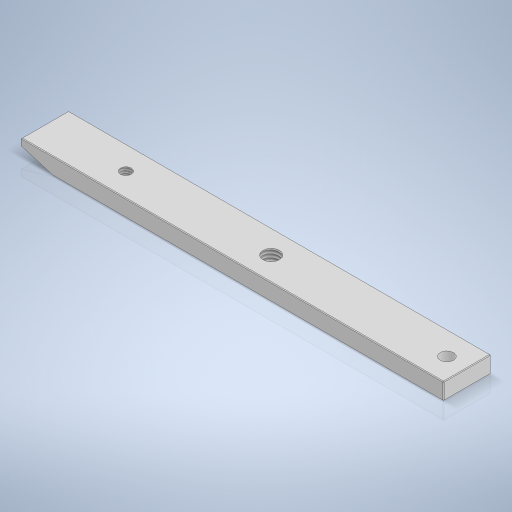
# Autodesk Inventor part: 112
Saved by Autodesk Inventor 2024 (Build 280153000, 153)
## iProperties
Created: 2024-06-07
Part Number: 112
Material: Generisch
Document SubType Name: Modeling
Designer: ffogue
Density: 1 g/cm^3
Appearance: Vorgabe
Author: ffogue
Autodesk Inventor part; units mm, degrees
ref_plane "YZ Plane" through (0, 0, 0) normal (1, 0, 0) x (0, 1, 0)
ref_plane "XZ Plane" through (0, 0, 0) normal (0, 1, 0) x (-1, 0, 0)
ref_plane "XY Plane" through (0, 0, 0) normal (0, 0, 1) x (1, 0, 0)
sketch "Skizze1" plane through (0, 0, 0) normal (0, 1, 0) x (-1, 0, 0)
  line L0 (0, 3) -> (0, 5)
  line L1 (0, 5) -> (-125, 5)
  line L2 (-125, 5) -> (-125, 0)
  line L3 (-125, 0) -> (-10, 0)
  line L4 (-10, 0) -> (0, 3)
  point P0 (0, 0)
  dimension "d0" = 10
  dimension "d1" = 2
  dimension "d2" = 125
  dimension "d3" = 5
  constraints: 10 end point, 3 perpendicular, 1 horizontal alignment, 1 vertical, 1 vertical alignment
  measures "d0" horizontal distance of L3.end L0.start
  measures "d1" distance of L0.start L0.end
  measures "d2" distance of L0.end L1.end
  measures "d3" distance between parallel lines of L3 L1
extrude "Extrusion1" add sketch "Skizze1" along normal blind 14
sketch "Skizze2" plane through (0, 0, 5) normal (0, 0, 1) x (1, 0, 0)
  line L0 (0, 0) -> (0, 14) projected
  point P0 (24, 7)
  point P1 (0, 7)
  dimension "d13" = 24
  constraints: 1 horizontal alignment, 1 midpoint
  measures "d13" distance from line of point (24, 7) L0
hole "Bohrung1" at (24, 7, 5) direction (0, 0, -1) diameter 3.242 depth 5 thread size "M4x0.7" class "6H" standard "ISO Metric profile"
sketch "Skizze3" plane through (0, 0, 5) normal (0, 0, 1) x (1, 0, 0)
  circle A0 centre (24, 7) radius 1.621 projected
  line L0 (0, 0) -> (0, 14) projected
  point P0 (67, 7)
  point P1 (0, 7)
  dimension "d21" = 43
  constraints: 1 horizontal alignment, 1 midpoint
  measures "d21" distance of point (67, 7) A0.centre
hole "Bohrung2" at (67, 7, 5) direction (0, 0, -1) diameter 4.917 end through all thread size "M6x1" class "6H" standard "ISO Metric profile"
sketch "Skizze4" plane through (0, 0, 5) normal (0, 0, 1) x (1, 0, 0)
  line L0 (0, 0) -> (0, 14) projected
  circle A0 centre (67, 7) radius 2.4585 projected
  line L1 (125, 0) -> (125, 14) projected
  point P0 (119, 7)
  point P1 (0, 7)
  point P2 (125, 7)
  dimension "d29" = 52
  dimension "d30" = 6
  constraints: 2 midpoint, 1 horizontal alignment
  measures "d29" distance of point (119, 7) A0.centre
  measures "d30" distance of point (125, 7) point (119, 7)
hole "Bohrung3" at (119, 7, 5) direction (0, 0, -1) diameter 4 end through all
chamfer "Fasen1" distance 0.2 angle 45 9 edges at (62.5, 0, 5) (62.5, 14, 5) (125, 7, 5) (125, 0, 2.5) (67.5, 0, 0) (125, 7, 0) (125, 14, 2.5) (67.5, 14, 0) (0, 7, 5)
